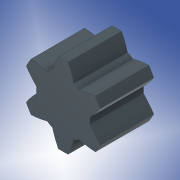
# Autodesk Inventor part: SJ012
Saved by Autodesk Inventor 2017 SP1 (Build 210196100, 196)
## iProperties
Created: 2017-07-04
Part Number: SJ012
Material: ABS Plastic
Document SubType Name: Modeling
Designer: Zach
Density: 1.06 g/cm^3
Appearance: CR Dark Blue
Author: Zach
Autodesk Inventor part; units mm, degrees
ref_plane "YZ Plane" through (0, 0, 0) normal (1, 0, 0) x (0, 1, 0)
ref_plane "XZ Plane" through (0, 0, 0) normal (0, 1, 0) x (-1, 0, 0)
ref_plane "XY Plane" through (0, 0, 0) normal (0, 0, 1) x (1, 0, 0)
sketch "Sketch1" plane through (0, 0, 0) normal (0, 0, 1) x (1, 0, 0)
  circle A0 centre (0, 0) radius 5
  dimension "d0" = 10
  constraints: 1 centre point, 1 coincident
  measures "d0" diameter of A0
extrude "Extrusion1" add sketch "Sketch1" along normal blind 10
sketch "Sketch3" plane through (0, 0, 10) normal (0, 0, 1) x (1, 0, 0)
  circle A0 centre (0, 0) radius 5 construction
  arc A1 (-2, -4.5826) -> (-0.9, -7.4458) centre (12.4788, -0.663) ccw
  arc A2 (0.9, -7.4458) -> (2, -4.5826) centre (-12.4788, -0.663) ccw
  arc A3 (-2, -4.5826) -> (2, -4.5826) centre (0, 0) ccw
  arc A4 (-0.9, -7.4458) -> (0.9, -7.4458) centre (0, 12.5339) ccw
  circle A5 centre (0, 0) radius 7.5 construction
  line L0 (0, 0) -> (0, -8.6797) construction
  arc A6 (2.9686, -4.0233) -> (5.9983, -4.5023) centre (6.8136, 10.4755) ccw
  arc A7 (2.9686, -4.0233) -> (4.9686, -0.5592) centre (0, 0) ccw
  arc A8 (6.8983, -2.9435) -> (4.9686, -0.5592) centre (-5.6653, -11.1385) ccw
  arc A9 (5.9983, -4.5023) -> (6.8983, -2.9435) centre (-10.8547, 6.267) ccw
  arc A10 (4.9686, 0.5592) -> (6.8983, 2.9435) centre (-5.6653, 11.1385) ccw
  arc A11 (4.9686, 0.5592) -> (2.9686, 4.0233) centre (0, 0) ccw
  arc A12 (5.9983, 4.5023) -> (2.9686, 4.0233) centre (6.8136, -10.4755) ccw
  arc A13 (6.8983, 2.9435) -> (5.9983, 4.5023) centre (-10.8547, -6.267) ccw
  arc A14 (2, 4.5826) -> (0.9, 7.4458) centre (-12.4788, 0.663) ccw
  arc A15 (2, 4.5826) -> (-2, 4.5826) centre (0, 0) ccw
  arc A16 (-0.9, 7.4458) -> (-2, 4.5826) centre (12.4788, 0.663) ccw
  arc A17 (0.9, 7.4458) -> (-0.9, 7.4458) centre (0, -12.5339) ccw
  arc A18 (-2.9686, 4.0233) -> (-5.9983, 4.5023) centre (-6.8136, -10.4755) ccw
  arc A19 (-2.9686, 4.0233) -> (-4.9686, 0.5592) centre (0, 0) ccw
  arc A20 (-6.8983, 2.9435) -> (-4.9686, 0.5592) centre (5.6653, 11.1385) ccw
  arc A21 (-5.9983, 4.5023) -> (-6.8983, 2.9435) centre (10.8547, -6.267) ccw
  arc A22 (-4.9686, -0.5592) -> (-6.8983, -2.9435) centre (5.6653, -11.1385) ccw
  arc A23 (-4.9686, -0.5592) -> (-2.9686, -4.0233) centre (0, 0) ccw
  arc A24 (-5.9983, -4.5023) -> (-2.9686, -4.0233) centre (-6.8136, 10.4755) ccw
  arc A25 (-6.8983, -2.9435) -> (-5.9983, -4.5023) centre (10.8547, 6.267) ccw
  point P0 (0, -7.4661)
  point P1 (0, -5)
  point P2 (4.3301, -2.5)
  point P3 (6.4658, -3.733)
  point P4 (4.3301, 2.5)
  point P5 (6.4658, 3.733)
  point P6 (0, 5)
  point P7 (0, 7.4661)
  point P8 (-4.3301, 2.5)
  point P9 (-6.4658, 3.733)
  point P10 (-4.3301, -2.5)
  point P11 (-6.4658, -3.733)
  dimension "d12" = 15
  dimension "d13" = 15
  dimension "d14" = 1.8
  dimension "d15" = 4
  dimension "d16" = 20
  dimension "d17" = 15
  dimension "d20" = 360
  constraints: 54 point on circle, 25 centre point, 2 end point, 2 point on line, 1 coincident, 1 concentric, 1 vertical, 85 other
  measures "d12" radius of A1
  measures "d13" radius of A2
  measures "d14" distance of A2.start A1.end
  measures "d15" distance of A0.end A0.start
  measures "d16" radius of A4
  measures "d17" diameter of A5
extrude "Extrusion2" add sketch "Sketch3" against normal blind 10
body "Solid1"
